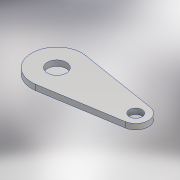
# Autodesk Inventor part: plate
Saved by Autodesk Inventor 2018.2 (Build 222227000, 227)
## iProperties
Created: 2017-12-11
Part Number: plate
Material: アルミニウム 6061
Document SubType Name: Modeling
Designer: kuwano
Density: 2.7 g/cm^3
Appearance: アルミニウム - フラット
Mass: 14.6918 g
Surface Area: 39.4766 cm^2
Volume: 5.4414 cm^3
Author: kuwano
Autodesk Inventor part; units mm, degrees
ref_plane "YZ Plane" through (0, 0, 0) normal (1, 0, 0) x (0, 1, 0)
ref_plane "XZ Plane" through (0, 0, 0) normal (0, 1, 0) x (-1, 0, 0)
ref_plane "XY Plane" through (0, 0, 0) normal (0, 0, 1) x (1, 0, 0)
sketch "スケッチ1" plane through (0, 0, 0) normal (0, 0, 1) x (1, 0, 0)
  circle A0 centre (0, 0) radius 6
  circle A1 centre (50, 0) radius 4
  arc A2 (2.56, 15.7939) -> (2.56, -15.7939) centre (0, 0) ccw
  line L0 (2.56, 15.7939) -> (100, 0)
  line L1 (100, 0) -> (2.56, -15.7939)
  line L2 (-39.2, 0) -> (123.2, 0) projected
  dimension "d0" = 50
  dimension "d1" = 12
  dimension "d2" = 10
  dimension "d3" = 8
  dimension "d4" = 8
  dimension "d5" = 8
  constraints: 4 end point, 3 centre point, 2 coincident, 2 point on circle, 2 tangent, 1 point on line
  measures "d0" distance of A1.centre point (0, 0)
  measures "d1" diameter of A0
  measures "d2" radial gap between concentric circles of A0 A2
  measures "d3" diameter of A1
  measures "d4" distance from line of L0 A1.centre
  measures "d5" distance from line of L1 A1.centre
extrude "押し出し1" add sketch "スケッチ1" along normal mid plane 3.5 contours L2 A1 L1 A2 A0 | A0 L2 A2 L0 A1
fillet "フィレット1" radius 8 1 edges at (100, 0, 0)
equation "\"d5\" = d4"
